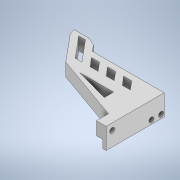
# Autodesk Inventor part: pinza fija
Saved by Autodesk Inventor 2021 (Build 250183000, 183)
## iProperties
Created: 2022-04-17
Part Number: pinza fija
Material: Genérico
Document SubType Name: Modeling
Designer: orgyn
Density: 1 g/cm^3
Appearance: Valor por defecto
Author: orgyn
Autodesk Inventor part; units mm, degrees
ref_plane "YZ Plane" through (0, 0, 0) normal (1, 0, 0) x (0, 1, 0)
ref_plane "XZ Plane" through (0, 0, 0) normal (0, 1, 0) x (-1, 0, 0)
ref_plane "XY Plane" through (0, 0, 0) normal (0, 0, 1) x (1, 0, 0)
sketch "Boceto1" plane through (0, 0, 0) normal (0, 1, 0) x (-1, 0, 0)
  circle A0 centre (0, 0) radius 1.5
  circle A1 centre (0, 0) radius 3
  arc A2 (5.7446, 4) -> (0, -7) centre (0, 0) ccw
  line L0 (5.7446, 4) -> (35, 4)
  line L1 (35, 4) -> (50, -14)
  line L2 (0, -10) -> (20, -10)
  line L3 (20, -10) -> (20, -16)
  line L4 (20, -16) -> (50, -16)
  line L5 (50, -16) -> (50, -14)
  line L6 (50, -16) -> (50, -16.5)
  line L7 (50, -16.5) -> (49.0807, -16.5)
  line L8 (0, -7) -> (0, -10)
  point P0 (0, 4)
  dimension "d1" = 6
  dimension "d8" = 6
  dimension "d9" = 0.5
  constraints: 18 end point, 3 centre point, 3 coincident, 2 perpendicular, 2 point on circle, 1 horizontal, 1 point on line, 1 vertical
  measures "d1" diameter of A1
  measures "d8" distance of L2.end L3.end
  measures "d9" distance of L4.end L6.end
extrude "Extrusión1" add sketch "Boceto1" along normal blind 8 contours A1 | L0 L1 L5 L4 L3 L2 L8 A2
sketch "Boceto2" plane through (0, 8, 0) normal (0, 1, 0) x (1, 0, 0)
  circle A0 centre (0, 0) radius 3
  dimension "d12" = 6
  constraints: 1 centre point, 1 coincident
  measures "d12" diameter of A0
extrude "Extrusión2" cut sketch "Boceto2" against normal blind 4
sketch "Boceto3" plane through (0, 0, 0) normal (0, -1, 0) x (1, 0, 0)
  line L0 (0, 0) -> (7, 0)
  arc A0 (0, -7) -> (-5.7446, 4) centre (0, 0) ccw projected
  line L1 (7, 0) -> (12, 0)
  line L2 (12, 0) -> (12, -10)
  line L3 (0, -10) -> (-20, -10) projected
  line L4 (12, -10) -> (0, -10)
  line L5 (12, 0) -> (12, 7.5855)
  line L6 (-35, 4) -> (-5.7446, 4) projected
  line L7 (-5.7446, 4) -> (12, 4)
  line L8 (0, -10) -> (0, 4)
  point P0 (0, -7)
  dimension "d15" = 5
  constraints: 14 end point, 4 perpendicular, 3 point on line, 1 horizontal, 1 point on circle, 1 vertical
  measures "d15" distance of L0.end L1.end
extrude "Extrusión3" add sketch "Boceto3" against normal blind 8 contours L1 L2 L4 L8 A0
sketch "Boceto4" plane through (12, 0, 0) normal (1, 0, 0) x (0, 0, -1)
  line L0 (10, 0) -> (0, 0) projected
  line L1 (0, 0) -> (0, -5)
  line L2 (0, -5) -> (10, -5)
  line L3 (10, -5) -> (10, 0)
  line L4 (10, 0) -> (0, 0)
  line L5 (10, -2.5) -> (0, -2.5)
  line L6 (10, -2.5) -> (8, -2.5)
  line L7 (0, -2.5) -> (2, -2.5)
  circle A0 centre (8, -2.5) radius 1.5
  circle A1 centre (2, -2.5) radius 1.5
  dimension "d18" = 5
  dimension "d19" = 2
  dimension "d20" = 2
  dimension "d21" = 3
  dimension "d22" = 3
  constraints: 14 end point, 3 perpendicular, 2 centre point, 2 coincident, 2 midpoint, 2 point on line, 1 vertical
  measures "d18" distance of L0.end L1.end
  measures "d19" distance of L5.start L6.end
  measures "d20" distance of L5.end L7.end
  measures "d21" diameter of A0
  measures "d22" diameter of A1
extrude "Extrusión4" add sketch "Boceto4" against normal blind 3 contours L3 L5 A0 A1 L1 L0 | L3 L2 L1 L5 A1 A0
sketch "Boceto5" plane through (0, 8, 0) normal (0, 1, 0) x (1, 0, 0)
  circle A0 centre (0, 0) radius 3
  circle A1 centre (0, 0) radius 1.5
  dimension "d25" = 3
  constraints: 2 centre point, 2 coincident
  measures "d25" diameter of A1
extrude "Extrusión5" add sketch "Boceto5" against normal blind 5
sketch "Boceto6" plane through (0, 0, 0) normal (0, -1, 0) x (1, 0, 0)
  line L0 (-50, -17) -> (-20, -17) projected
  line L1 (-50, -16) -> (-50, -14) projected
  line L2 (-50, -17) -> (-50, -16)
  line L3 (-50, -16.5) -> (-16.403, -16.5)
  line L4 (-20, -23) -> (-25, -23)
  line L5 (-5.7446, -37) -> (-35, -37) projected
  line L6 (-25, -23) -> (-25, -28)
  line L7 (-25, -37) -> (-25, -32)
  line L8 (-25, -32) -> (-5.7446, -32)
  line L9 (-5.7446, -32) -> (-5.7446, -27.061)
  line L10 (-25, -28) -> (-5.7446, -28)
  line L11 (-35, -37) -> (-30, -37)
  line L12 (-30, -37) -> (-30, -32)
  line L13 (-30, -32) -> (-25, -32)
  line L14 (-50, -19) -> (-50, -17) projected
  line L15 (-50, -19) -> (-45, -19)
  line L16 (-30, -37) -> (-45, -19)
  line L17 (-45, -19) -> (-40, -19)
  line L18 (-30, -32) -> (-40.8333, -19)
  line L19 (-40.8333, -19) -> (-25, -19)
  line L20 (-25, -19) -> (-25, -28)
  line L21 (-30, -32) -> (-34.1667, -32)
  line L22 (-40.8333, -19) -> (-35.8333, -19)
  line L23 (-35.8333, -19) -> (-25, -32)
  line L24 (-35.8333, -19) -> (-30.8333, -19)
  line L25 (-25, -32) -> (-20, -32)
  line L26 (-20, -32) -> (-30.8333, -19)
  line L27 (-30, 4) -> (-45, -14)
  line L28 (-45, -14) -> (-40, -14)
  line L29 (-30, -1) -> (-40.8333, -14)
  line L30 (-30, -1) -> (-34.1667, -1)
  line L31 (-35.8333, -14) -> (-25, -1)
  line L32 (-35.8333, -14) -> (-30.8333, -14)
  line L33 (-25, -1) -> (-20, -1)
  line L34 (-20, -1) -> (-30.8333, -14)
  point P0 (0, 0)
  dimension "d28" = 5
  dimension "d29" = 5
  dimension "d30" = 5
  dimension "d31" = 5
  dimension "d32" = 5
  dimension "d33" = 5
  dimension "d34" = 5
  dimension "d35" = 5
  dimension "d36" = 5
  constraints: 62 end point, 12 point on line, 10 symmetric about line, 5 perpendicular, 3 horizontal, 3 parallel, 2 vertical, 1 collinear, 1 midpoint
  measures "d28" distance of L4.start L4.end
  measures "d29" distance of L4.end L6.end
  measures "d30" distance of L7.start L7.end
  measures "d31" distance of L5.end L11.end
  measures "d32" distance of L14.start L15.end
  measures "d33" distance of L15.end L17.end
  measures "d34" distance of L18.end L22.end
  measures "d35" distance of L22.end L24.end
  measures "d36" distance of L7.end L25.end
extrude "Extrusión6" cut sketch "Boceto6" against normal blind 10 contours L23 L19 L26 L6 L10 L8 | L21 L16 L17 L18 | L10 L6 L26 | L30 L29 L28 L27 | L31 L33 L34 L32
sketch "Boceto7" plane through (0, 0, 0) normal (0, -1, 0) x (1, 0, 0)
  line L0 (-35, 4) -> (-5.7446, 4) projected
  arc A0 (7, 0) -> (-5.7446, 4) centre (0, 0) ccw projected
  line L1 (-5.7446, 4) -> (7, 0)
  line L2 (7, 0) -> (8.04, 10.76)
  line L3 (8.04, 10.76) -> (-8.8935, 9.8507)
  line L4 (-8.8935, 9.8507) -> (-5.7446, 4)
  constraints: 8 end point
extrude "Extrusión7" cut sketch "Boceto7" against normal blind 10 contours L1 A0
sketch "Boceto8" plane through (0, 0, 0) normal (0, -1, 0) x (1, 0, 0)
  circle A0 centre (0, 0) radius 1.5
  constraints: 1 centre point, 1 coincident
extrude "Extrusión8" add sketch "Boceto8" against normal blind 8
fillet "Empalme1" radius 2 2 edges at (9, -5, -5) (9, 0, -5)
chamfer "Chaflán1" distance 2 angle 45 1 edges at (-50, 4, -14)
sketch "Boceto9" plane through (0, 0, 0) normal (0, -1, 0) x (1, 0, 0)
  circle A0 centre (0, -33) radius 1.5 projected
  circle A1 centre (0, -33) radius 3
  point P0 (0, 0)
  dimension "d47" = 6
  constraints: 1 centre point, 1 coincident
  measures "d47" diameter of A1
extrude "Extrusión9" cut sketch "Boceto9" against normal blind 4
sketch "Boceto10" plane through (0, 8, 0) normal (0, 1, 0) x (1, 0, 0)
  circle A0 centre (0, 33) radius 1.5 projected
  circle A1 centre (0, 33) radius 6
  line L0 (0, 33) -> (-19, 33)
  line L1 (0, 33) -> (0, 37.5)
  line L2 (0, 37.5) -> (-19, 37.5)
  line L3 (-19, 37.5) -> (-19, 28.5)
  line L4 (-19, 28.5) -> (0, 28.5)
  line L5 (-19, 33) -> (-16, 33)
  circle A2 centre (-16, 33) radius 3
  circle A3 centre (-16, 33) radius 3
  line L6 (-16, 36) -> (-3.9686, 37.5)
  line L7 (-16, 33) -> (-16, 30)
  line L8 (-16, 30) -> (-3.9686, 28.5)
  point P0 (0, 0)
  dimension "d50" = 12
  dimension "d51" = 19
  dimension "d52" = 4.5
  dimension "d53" = 9
  dimension "d54" = 3
  constraints: 18 end point, 4 point on circle, 4 point on line, 3 coincident, 3 perpendicular, 2 centre point, 1 horizontal, 1 vertical, 4 other
  measures "d50" diameter of A1
  measures "d51" distance of L0.start L0.end
  measures "d52" distance of L0.start L1.end
  measures "d53" distance of L2.end L3.end
  measures "d54" distance of L0.end L5.end
extrude "Extrusión10" cut sketch "Boceto10" against normal blind 2 contours A0 L1 L2 A1 L0 | A0 L0 A1 L2 L1 | L0 A2 L6 A1 | A1 L8 A2 L0 | A2 L7 L0 | L0 A2 | A2 L0 L7
sketch "Boceto12" plane through (0, 0, 0) normal (0, -1, 0) x (1, 0, 0)
  line L0 (12, -10) -> (-20, -10) projected
  line L1 (12, -10) -> (10, -10)
  line L2 (10, -10) -> (10, 61.6963)
  line L3 (10, 0) -> (10, 20)
  line L4 (-35, 4) -> (-5.7446, 4) projected
  line L5 (10, 20) -> (-35, 4)
  line L6 (7, 0) -> (-5.7446, 4) projected
  line L7 (-35, 4) -> (-5.7446, 4)
  line L8 (-5.7446, 4) -> (7, 0)
  line L9 (7, 0) -> (10, 0)
  line L10 (-35, 4) -> (-30, 4)
  line L11 (10, 20) -> (10, 15)
  line L12 (10, 15) -> (-30, 4)
  line L13 (-30, 4) -> (-25, 4)
  line L14 (-25, 4) -> (-25, 5.375)
  line L15 (-25, 5.375) -> (-4, 5.375)
  line L16 (-4, 5.375) -> (-4, 11.15)
  line L17 (-15.4357, -10) -> (-15.4357, -5)
  line L18 (-15.4357, -5) -> (-15.4357, 0)
  line L19 (-15.4357, 0) -> (-1.6825, -0.962)
  line L20 (-15.4357, 0) -> (0, 0)
  line L21 (0, 0) -> (0, -5)
  line L22 (0, -5) -> (-15.4357, -5)
  dimension "d57" = 2
  dimension "d58" = 20
  dimension "d59" = 5
  dimension "d60" = 5
  dimension "d61" = 5
  dimension "d64" = 5
  constraints: 40 end point, 10 point on line, 5 perpendicular, 2 horizontal, 2 parallel, 1 vertical
  measures "d57" distance of L0.start L1.end
  measures "d58" distance of L3.start L3.end
  measures "d59" distance of L4.start L10.end
  measures "d60" distance of L3.end L11.end
  measures "d61" distance of L10.end L13.end
  measures "d64" distance of L17.start L17.end
extrude "Extrusión11" add sketch "Boceto12" against normal blind 8 contours L9 L6 L4 L14 L15 L16 L12 L2 | L12 L4 L5 L2 | L14 L4 L12 | L18 L20 L21 L22
sketch "Boceto14" plane through (0, 0, 0) normal (0, -1, 0) x (1, 0, 0)
  line L0 (-40.8333, -14) -> (-30, -1) projected
  line L1 (-35.8333, -14) -> (-30.8333, -14) projected
  line L2 (-40.8333, -14) -> (-35.8333, -14)
  line L3 (-35.8333, -14) -> (-38.3333, -14)
  line L4 (-25, -1) -> (-35.8333, -14) projected
  line L5 (-35.8333, -14) -> (-29.4226, -6.3071)
  line L6 (-34.4226, -6.3071) -> (-29.4226, -6.3071)
  line L7 (-29.4226, -6.3071) -> (-20, -6.3071)
  line L8 (-20, -10) -> (7, -10) projected
  line L9 (-20, -6.3071) -> (-20, -10)
  line L10 (-40.8333, -14) -> (-40.8333, -16)
  line L11 (-20, -16) -> (-50, -16) projected
  line L12 (-20, -10) -> (-20, -16) projected
  line L13 (-40.8333, -16) -> (-20, -16)
  line L14 (-20, -16) -> (-20, -10)
  line L15 (-35.8333, -14) -> (-30.8333, -14)
  line L16 (-30.8333, -14) -> (-20, -1) projected
  line L17 (-24.4226, -6.3071) -> (-30.8333, -14)
  line L18 (-35.8333, -14) -> (-40.8333, -16)
  line L19 (-50, -16) -> (-50, -17)
  line L20 (-50, -16.5) -> (-40.8333, -16.5)
  line L21 (-40.8333, -19) -> (-30, -32)
  line L22 (-35.8333, -19) -> (-30.8333, -19)
  line L23 (-40.8333, -19) -> (-35.8333, -19)
  line L24 (-35.8333, -19) -> (-38.3333, -19)
  line L25 (-25, -32) -> (-35.8333, -19)
  line L26 (-35.8333, -19) -> (-29.4226, -26.6929)
  line L27 (-34.4226, -26.6929) -> (-29.4226, -26.6929)
  line L28 (-29.4226, -26.6929) -> (-20, -26.6929)
  line L29 (-20, -26.6929) -> (-20, -23)
  line L30 (-40.8333, -19) -> (-40.8333, -17)
  line L31 (-20, -23) -> (-20, -17)
  line L32 (-40.8333, -17) -> (-20, -17)
  line L33 (-20, -17) -> (-20, -23)
  line L34 (-35.8333, -19) -> (-30.8333, -19)
  line L35 (-30.8333, -19) -> (-20, -32)
  line L36 (-24.4226, -26.6929) -> (-30.8333, -19)
  line L37 (-35.8333, -19) -> (-40.8333, -17)
  point P0 (0, 0)
  constraints: 62 end point, 15 point on line, 15 symmetric about line, 4 horizontal, 2 collinear, 2 midpoint, 1 perpendicular, 1 vertical
extrude "Extrusión13" cut sketch "Boceto14" against normal blind 8 contours L18 L1 L16 L7 L9 L12 L11 | L32 L31 L29 L28 L35 L22 L37
sketch "Boceto15" plane through (0, 0, 0) normal (0, -1, 0) x (1, 0, 0)
  line L0 (-20, -6.3071) -> (-24.4226, -6.3071) projected
  line L1 (-20, -6.3071) -> (-29.4226, -6.3071)
  line L2 (-35.8333, -14) -> (-25, -1) projected
  line L3 (-20, -10) -> (-20, -6.3071) projected
  line L4 (-20, -10) -> (-32.5381, -10)
  line L5 (-32.5381, -10) -> (-29.4226, -6.3071)
  line L6 (-50, -17) -> (-40.8333, -17) projected
  line L7 (-40.8333, -16) -> (-50, -16) projected
  line L8 (-50, -17) -> (-50, -16)
  line L9 (-50, -16.5) -> (-36.6527, -16.5)
  point P0 (0, 0)
  point P1 (-32.5, -10)
  constraints: 10 end point, 3 horizontal, 1 midpoint, 1 point on line, 1 vertical
extrude "Extrusión14" add sketch "Boceto15" against normal blind 8 contours L3 L4 L2 L1 L0
sketch "Boceto16" plane through (0, 0, 0) normal (0, -1, 0) x (1, 0, 0)
  line L0 (-29.4226, -26.6929) -> (-25, -32) projected
  line L1 (-25, -32) -> (-5.7446, -32)
  line L2 (-25, -1) -> (-20, -1) projected
  line L3 (-20, -1) -> (-15, -1)
  line L4 (-15, -1) -> (-10, -1)
  line L5 (-10, -1) -> (-5, -1)
  line L6 (-5, -1) -> (0, -1)
  line L7 (-20, -1) -> (-24.4226, -6.3071) projected
  line L8 (-24.4226, -6.3071) -> (-19.4226, -6.3071)
  line L9 (-19.4226, -6.3071) -> (-14.4226, -6.3071)
  line L10 (-14.4226, -6.3071) -> (-9.4226, -6.3071)
  line L11 (-9.4226, -6.3071) -> (-4.4226, -6.3071)
  line L12 (-25, -1) -> (-29.4226, -6.3071) projected
  line L13 (-19.4226, -6.3071) -> (-15, -1)
  line L14 (-14.4226, -6.3071) -> (-10, -1)
  line L15 (-9.4226, -6.3071) -> (-5, -1)
  line L16 (-4.4226, -6.3071) -> (0, -1)
  point P0 (0, 0)
  dimension "d72" = 5
  dimension "d73" = 5
  dimension "d74" = 5
  dimension "d75" = 5
  dimension "d76" = 5
  dimension "d77" = 5
  dimension "d78" = 5
  dimension "d79" = 5
  constraints: 26 end point, 6 point on line, 3 horizontal
  measures "d72" distance of L2.end L3.end
  measures "d73" distance of L3.end L4.end
  measures "d74" distance of L4.end L5.end
  measures "d75" distance of L5.end L6.end
  measures "d76" distance of L7.end L8.end
  measures "d77" distance of L8.end L9.end
  measures "d78" distance of L9.end L10.end
  measures "d79" distance of L10.end L11.end
extrude "Extrusión15" cut sketch "Boceto16" against normal blind 8 contours L4 L14 L9 L13 | L6 L16 L11 L15
sketch "Boceto17" plane through (10, 0, 20) normal (1, 0, 0) x (0, 0, -1)
  line L0 (0, 0) -> (0, 8) projected
  line L1 (20.8978, 8) -> (0, 8)
  line L2 (0, 8) -> (0, -14.2974)
  line L3 (20, 8) -> (20, -5) projected
  line L4 (20, -5) -> (0, -5)
  point P0 (20, 0)
  constraints: 6 end point, 2 perpendicular, 1 horizontal, 1 point on line
extrude "Extrusión16" add sketch "Boceto17" along normal blind 2
sketch "Boceto19" plane through (11, -5, -10) normal (0, -1, 0) x (1, 0, 0)
  line L0 (-1, 30) -> (-1, 10) projected
  line L1 (-1, 30) -> (-5, 30)
  line L2 (-5, 30) -> (-5, 25.9767)
  line L3 (-1, 30) -> (-46, 14) projected
  line L4 (-5, 28.5778) -> (-1, 30)
  line L5 (-1, 30) -> (-1, 36)
  line L6 (-1, 36) -> (1, 36)
  line L7 (1, 30) -> (1, 0) projected
  line L8 (1, 36) -> (1, 30)
  line L9 (-5, 30) -> (-5, 36)
  line L10 (-5, 36) -> (-1, 36)
  line L11 (-1, 30) -> (1, 30) projected
  line L12 (-1, 30) -> (1, 30)
  point P0 (-11, 10)
  dimension "d84" = 4
  dimension "d85" = 6
  constraints: 18 end point, 4 perpendicular, 2 collinear, 2 point on line, 2 vertical, 1 horizontal
  measures "d84" distance of L0.start L1.end
  measures "d85" distance of L0.start L5.end
extrude "Extrusión17" add sketch "Boceto19" against normal blind 13
sketch "Boceto20" plane through (0, 0, 0) normal (0, -1, 0) x (1, 0, 0)
  line L0 (10, 20) -> (10, 0) projected
  line L1 (10, 20) -> (5.8802, 18.5352)
  line L2 (6, 18.5778) -> (-35, 4) projected
  line L3 (5.8802, 18.5352) -> (5.8802, 28.5121)
  line L4 (10, 20) -> (10, 30.9812)
  line L5 (10, 30.9812) -> (5.8802, 28.5121)
  point P0 (0, 0)
  constraints: 8 end point, 2 vertical, 1 point on line
extrude "Extrusión18" cut sketch "Boceto20" along normal blind 13
sketch "Boceto21" plane through (6, 0, 26) normal (-1, 0, 0) x (0, 0, 1)
  line L0 (-7.4222, 0) -> (-22, 0) projected
  line L1 (-7.4222, 0) -> (-7.4222, 8)
  line L2 (-36, 8) -> (0, 8) projected
  line L3 (-7.4222, 0) -> (-0.2368, 0)
  line L4 (-7.4222, 0) -> (0, 0) projected
  line L5 (-7.4222, 0) -> (-7.4222, 8) projected
  line L6 (-3.7111, 0) -> (-3.7111, 8)
  line L7 (-7.4222, 8) -> (0, 8) projected
  line L8 (-7.4222, 4) -> (0, 4)
  circle A0 centre (-3.7111, 4) radius 1.5
  point P0 (-26, 0)
  dimension "d90" = 3
  constraints: 8 end point, 4 midpoint, 2 point on line, 1 centre point, 1 horizontal, 1 vertical
  measures "d90" diameter of A0
extrude "Extrusión19" cut sketch "Boceto21" against normal blind 13 contours A0 L6 L8 | L8 L6 A0 | L6 L8 A0 | L6 A0 L8
chamfer "Chaflán2" distance 1 angle 45 1 edges at (6, 4, 20.7889)
